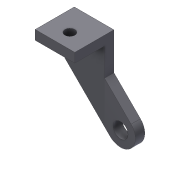
# Autodesk Inventor part: PWTR-0043
Saved by Autodesk Inventor 2020 (Build 240168000, 168)
## iProperties
Part Number: PWTR-0043
Document SubType Name: Modeling
Created: 2003-02-09
Designer: B. BOGAN
Material: Stainless Steel, 303
Density: 7.75 g/cm^3
Mass: 10.2686 g
Surface Area: 12.7032 cm^2
Volume: 1.32499 cm^3
Appearance: Steel
Vendor: Non-Design Specific
Control State: 0
Master: False
Checked Out: False
Shininess: 64.0
Length Units: 11269
Angle Units: 11279
Time Units: 11290
Mass Units: 11283
Length Display Precision: 3
Angle Display Precision: 2
Compacted: True
Density: 0.0
Volumn: 0.0
Area: 0.0
PropertySet Name: Model Information
Title: PITCH CONTROL ARM
Author: B. BOGAN
Revision Number: B
Autodesk Inventor part; units mm, degrees
ref_plane "YZ Plane" through (0, 0, 0) normal (1, 0, 0) x (0, 1, 0)
ref_plane "XZ Plane" through (0, 0, 0) normal (0, 1, 0) x (-1, 0, 0)
ref_plane "XY Plane" through (0, 0, 0) normal (0, 0, 1) x (1, 0, 0)
sketch "Sketch1" plane through (0, 0, 0) normal (0, 0, 1) x (1, 0, 0)
  line L0 (0, 0) -> (12.7, 0)
  line L1 (12.7, 0) -> (12.7, -11.9296)
  line L2 (0, 0) -> (0, -12.7)
  line L3 (0, -12.7) -> (14.4801, -27.1801)
  arc A0 (14.4801, -27.1801) -> (21.2153, -20.4449) centre (17.8477, -23.8125) ccw
  line L4 (21.2153, -20.4449) -> (12.7, -11.9296)
  dimension "d10" = 12.7
  dimension "d11" = 12.7
  dimension "d12" = 45
  dimension "d13" = 23.8125
  dimension "d14" = 4.7625
  constraints: 10 end point, 2 parallel, 2 point on circle, 2 tangent, 1 centre point, 1 coincident, 1 horizontal, 1 perpendicular
  measures "d10" distance between parallel lines of L1 L2
  measures "d11" distance from line of L2.end L0
  measures "d12" angle of L3 L2
  measures "d13" distance from line of A0.centre L0
  measures "d14" radius of A0
extrude "Extrusion1" add sketch "Sketch1" along normal blind 3
sketch "Sketch2" plane through (0, 0, 3) normal (0, 0, 1) x (1, 0, 0)
  line L0 (12.7, 0) -> (12.7, -11.9296) projected
  line L1 (0, 0) -> (12.7, 0) projected
  line L2 (0, -12.7) -> (0, 0) projected
  line L3 (0, -3) -> (12.7, -3)
  dimension "d17" = 3
  constraints: 2 end point, 2 point on line, 1 perpendicular
  measures "d17" distance between parallel lines of L3 L1
extrude "Extrusion2" add sketch "Sketch2" along normal blind 9.525
sketch "Sketch3" plane through (0, 0, 0) normal (0, 1, 0) x (1, 0, 0)
  line L0 (0, 0) -> (0, -12.525) projected
  line L1 (0, -12.525) -> (12.7, -12.525) projected
  point P0 (6.35, -7.7625)
  dimension "d20" = 4.7625
  dimension "d21" = 6.35
  measures "d20" distance from line of point (6.35, -7.762) L1
  measures "d21" distance from line of point (6.35, -7.762) L0
hole "Hole1" at (6.35, 0, 7.7625) direction (0, -1, 0) diameter 3.175 end through all
sketch "Sketch4" plane through (0, 0, 0) normal (0, 0, -1) x (-1, 0, 0)
  arc A0 (-21.2153, -20.4449) -> (-14.4801, -27.1801) centre (-17.8477, -23.8125) ccw projected
hole "Hole2" at (17.8477, -23.8125, 0) direction (0, 0, 1) diameter 4.826 end through all
body "Solid1"
